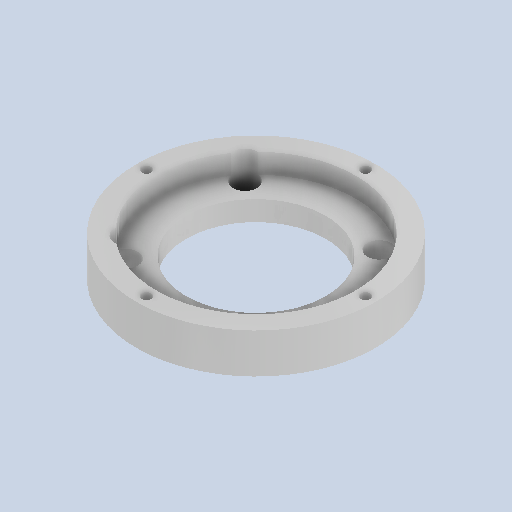
# Autodesk Inventor part: Placeholderjointouterring
Saved by Autodesk Inventor 2025.4 (Build 294407000, 407)
## iProperties
Created: 2026-03-22
Part Number: Placeholderjointouterring
Material: Aluminum 6061-AHC
Document SubType Name: Modeling
Designer: hp
Density: 2.7 g/cm^3
Appearance: Aluminum - Dark
Author: hp
Autodesk Inventor part; units mm, degrees
ref_plane "YZ Plane" through (0, 0, 0) normal (1, 0, 0) x (0, 1, 0)
ref_plane "XZ Plane" through (0, 0, 0) normal (0, 1, 0) x (-1, 0, 0)
ref_plane "XY Plane" through (0, 0, 0) normal (0, 0, 1) x (1, 0, 0)
sketch "Sketch1" plane through (0, 0, 0) normal (0, 1, 0) x (-1, 0, 0)
  circle A0 centre (0, 0) radius 25
  circle A1 centre (0, 0) radius 30
  circle A2 centre (0, 0) radius 17.5
  line L0 (0, 0) -> (25, 0) construction
  circle A3 centre (17.6777, -17.6777) radius 2
  circle A4 centre (17.6777, 17.6777) radius 2
  circle A5 centre (-17.6777, 17.6777) radius 2
  circle A6 centre (-17.6777, -17.6777) radius 2
  point P0 (0, -27.5)
  point P1 (0, -27.5)
  point P2 (27.5, 0)
  point P3 (-27.5, 0)
  point P4 (0, 27.5)
  dimension "d0" = 50
  dimension "d1" = 60
  dimension "d17" = 27.5
  dimension "d18" = 27.5
  dimension "d19" = 27.5
  dimension "d20" = 27.5
  dimension "d28" = 35
  dimension "d30" = 4
  dimension "d33" = 360
  constraints: 7 centre point, 4 coincident, 2 end point, 1 horizontal, 9 other
  measures "d0" diameter of A0
  measures "d1" diameter of A1
  measures "d17" distance of point (0, 0) point (27.5, 0)
  measures "d18" distance of point (-27.5, 0) point (0, 0)
  measures "d19" distance of point (0, 0) point (0, 27.5)
  measures "d20" distance of point (0, -27.5) point (0, 0)
  measures "d28" diameter of A2
  measures "d30" diameter of A3
extrude "Extrusion1" add sketch "Sketch1" along normal blind 5 contours A0 A4 | A3 A0 | A0 A5 | A6 A0 | A1 picked at (18.1752, 18.1125) picked at (18.1752, -18.1125) picked at (-18.083, 18.1995) picked at (-18.083, -18.1995)
extrude "Extrusion2" add sketch "Sketch1" against normal blind 5 contours A0 A3 A6 A5 A4 | A4 A0 | A0 A4 | A3 A0 | A0 A3 | A5 A0 | A0 A5 | A6 A0 | A0 A6 | A1
hole "Hole2" at (0, 0, -27.5) at (-27.5, 0, 0) at (27.5, 0, 0) at (0, 0, 27.5) direction (0, 1, 0) diameter 2.45 end through all both
sketch "Sketch3" plane through (0, -5, 0) normal (0, -1, 0) x (1, 0, 0)
  circle A0 centre (16.0335, 14.9787) radius 3
  circle A1 centre (-15.7294, 16.8799) radius 3
  circle A2 centre (-17.6307, -14.8831) radius 3
  circle A3 centre (14.1323, -16.7843) radius 3
  point P0 (0, 0)
  constraints: 4 centre point, 8 other
extrude "Extrusion4" cut sketch "Sketch3" against normal blind 10
body "Solid1"
